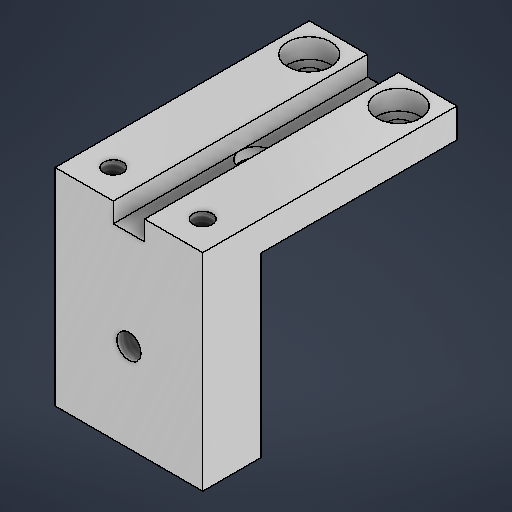
# Autodesk Inventor part: Bearing Sled
Saved by Autodesk Inventor 2026 (Build 300175050, 175E)
## iProperties
Created: 2025-05-26
Part Number: Bearing Sled
Material: Aluminum 6061
Document SubType Name: Modeling
Designer: Joshua Eah
Density: 2.7 g/cm^3
Appearance: Aluminum - Flat
Author: Joshua Eah
Autodesk Inventor part; units mm, degrees
ref_plane "YZ Plane" through (0, 0, 0) normal (1, 0, 0) x (0, 1, 0)
ref_plane "XZ Plane" through (0, 0, 0) normal (0, 1, 0) x (-1, 0, 0)
ref_plane "XY Plane" through (0, 0, 0) normal (0, 0, 1) x (1, 0, 0)
sketch "Sketch1" plane through (0, 0, 0) normal (0, 1, 0) x (-1, 0, 0)
  line L0 (0, 0) -> (-15, 0)
  line L1 (-15, 0) -> (-15, -25.825)
  line L2 (-15, -25.825) -> (0, -25.825)
  line L3 (0, -25.825) -> (0, 0)
  line L4 (-7.5, -25.825) -> (-7.5, 0) construction
  circle A0 centre (-7.5, -12.9125) radius 1.5
  line L5 (-15, -5.9125) -> (0, -5.9125)
  line L6 (0, -5.9125) -> (0, -19.9125)
  line L7 (0, -19.9125) -> (-15, -19.9125)
  line L8 (-15, -19.9125) -> (-15, -5.9125)
  line L9 (-15, -5.9125) -> (0, -19.9125) construction
  line L10 (0, -5.9125) -> (-15, -19.9125) construction
  circle A1 centre (-2.9563, -22.8688) radius 1
  circle A2 centre (-12.0437, -22.8688) radius 1
  circle A3 centre (-2.9563, -2.9563) radius 1
  circle A4 centre (-12.0438, -2.9563) radius 1
  line L11 (-5.9125, -25.825) -> (-9.0875, -25.825)
  line L12 (-9.0875, -25.825) -> (-9.0875, 0)
  line L13 (-9.0875, 0) -> (-5.9125, 0)
  line L14 (-5.9125, 0) -> (-5.9125, -25.825)
  line L15 (-5.9125, -25.825) -> (-9.0875, 0) construction
  line L16 (-9.0875, -25.825) -> (-5.9125, 0) construction
  point P0 (-15, -19.9125)
  point P1 (-15, -5.9125)
  point P2 (0, -5.9125)
  point P3 (-5.9125, -25.825)
  point P4 (-9.0875, 0)
  dimension "d0" = 15
  dimension "d2" = 3
  dimension "d3" = 12.9125
  dimension "d4" = 14
  dimension "d5" = 2
  dimension "d6" = 2.9562
  dimension "d7" = 2.9562
  dimension "d8" = 2.9562
  dimension "d9" = 2
  dimension "d11" = 2.9562
  dimension "d12" = 2.9562
  dimension "d13" = 2.9562
  dimension "d25" = 5.9125
  dimension "d68" = 3.175
  dimension "d81" = 25.825
  constraints: 34 end point, 7 midpoint, 6 parallel, 5 centre point, 3 horizontal, 3 perpendicular, 2 equal radius, 2 horizontal alignment, 2 point on line
  measures "d0" distance of L2.end L1.end
  measures "d2" diameter of A0
  measures "d3" distance from line of L2 A0.centre
  measures "d4" distance of L5.end L6.end
  measures "d5" diameter of A1
  measures "d6" distance from line of L2 A1.centre
  measures "d7" distance from line of A1.centre L3
  measures "d8" distance from line of L1 A2.centre
  measures "d9" diameter of A3
  measures "d11" distance from line of A3.centre L0
  measures "d12" distance from line of A3.centre L3
  measures "d13" distance from line of A4.centre L1
  measures "d25" distance between parallel lines of L5 L0
  measures "d68" distance of L12.end L13.end
  measures "d81" distance between parallel lines of L0 L2
extrude "Extrusion1" add sketch "Sketch1" against normal blind 3 contours L3 L5 L14 L0 | L14 L5 L12 L0 | L3 L7 L14 L5 | L12 L5 L1 L0 | L14 L7 L12 L5 | L3 L2 L14 L7 | L12 L7 L1 L5 | L14 L2 L12 L7 | L12 L2 L1 L7 | A0 | A1 | A2 | A3 | A4
extrude "Extrusion2" add sketch "Sketch1" against normal blind 21 contours L3 L5 L14 L0 | L14 L5 L12 L0 | L12 L5 L1 L0 | A3 | A4
hole "Hole3" at (2.9563, 0, -22.8688) at (12.0437, 0, -22.8688) direction (0, -1, 0) diameter 2.3876 end through all counterbore diameter 4.3942 counterbore depth 2 clearance for "Socket Head Cap Screw" size "M2" standard "Ansi Metric M Profile"
extrude "Extrusion3" cut sketch "Sketch1" against normal blind 2 contours L14 L5 L12 L0 | L14 L7 L12 L5 | L14 L2 L12 L7 | A0
sketch "Sketch3" plane through (0, -21, 0) normal (0, -1, 0) x (1, 0, 0)
  circle A0 centre (12.0437, -2.9563) radius 1
  circle A1 centre (2.9563, -2.9563) radius 1
  line L0 (15, 0) -> (0, 0) projected
  line L1 (15, -5.9125) -> (15, 0) projected
  line L2 (0, 0) -> (0, -5.9125) projected
  dimension "d44" = 2
  dimension "d45" = 2.9562
  dimension "d46" = 2.9562
  dimension "d47" = 2.9562
  constraints: 2 centre point, 1 equal radius, 1 horizontal alignment
  measures "d44" diameter of A0
  measures "d45" distance from line of L0 A0.centre
  measures "d46" distance from line of L1 A0.centre
  measures "d47" distance from line of L2 A1.centre
hole "Hole4" at (12.0437, -21, -2.9563) at (2.9563, -21, -2.9563) direction (0, 1, 0) diameter 1.9406 end through all thread size "3-48 UNC" class "2B" standard "ANSI Unified Screw Threads"
sketch "Sketch4" plane through (0, -3, 0) normal (0, -1, 0) x (1, 0, 0)
  circle A0 centre (7.5, -12.9125) radius 1.5
  point P0 (0, 0)
  dimension "d60" = 3
  constraints: 1 centre point, 1 coincident
  measures "d60" diameter of A0
hole "Hole5" at (7.5, -3, -12.9125) direction (0, 1, 0) diameter 3.2004 depth 1 clearance for "Socket Head Cap Screw" size "M3" standard "Ansi Metric M Profile"
sketch "Sketch5" plane through (0, -21, 0) normal (0, 0, 1) x (1, 0, 0)
  circle A0 centre (7.5, 9) radius 1.5
  line L0 (0, 21) -> (5.9125, 21) projected
  line L1 (0, 21) -> (0, 0) projected
  dimension "d71" = 3
  dimension "d72" = 12
  dimension "d73" = 7.5
  constraints: 1 centre point
  measures "d71" diameter of A0
  measures "d72" distance from line of L0 A0.centre
  measures "d73" distance from line of L1 A0.centre
hole "Hole6" at (7.5, -12, 0) direction (0, 0, -1) diameter 2.459 end through all thread size "M3x0.5" class "6H" standard "ANSI Metric M Profile"
equation "\"d3\" = 0.5 * d81"
equation "\"d6\" = d7"
equation "\"d7\" = -0.25 * d68 + 0.25 * d0"
equation "\"d8\" = d7"
equation "\"d11\" = d6"
equation "\"d12\" = d7"
equation "\"d13\" = d7"
equation "\"d25\" = 2 * d11"
equation "\"d45\" = d6"
equation "\"d46\" = d13"
equation "\"d47\" = d12"
body "Solid1"
